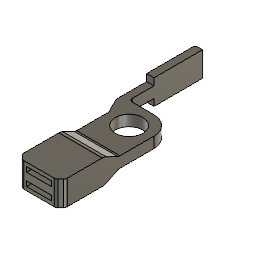
s.piece #1 (Autodesk Fusion 360 design; units mm, degrees)
part number: 2025-12-29-16-31-06-282
Autodesk Fusion 360 part; units mm, degrees
note: some values were not read from the file. Set by a fixed rule: which sketch regions a step uses.
sketch "Sketch1" plane through (0, 0, 0) normal (0, 0, 1) x (1, 0, 0)
  circle A0 centre (0, 0) radius 11
  line L0 (-17.5, -72.5) -> (17.5, -72.5)
  line L1 (17.5, -72.5) -> (17.5, 17.5)
  line L2 (17.5, 17.5) -> (-17.5, 17.5)
  line L3 (-17.5, 17.5) -> (-17.5, -72.5)
  line L4 (-17.5, 76.6964) -> (-17.5, 51.5115)
  line L5 (-17.5, 51.5115) -> (-17.5, 17.5)
  line L6 (-23.5, 76.6964) -> (-23.5, 13.1317)
  line L7 (-23.5, 13.1317) -> (-17.5, 1.0512)
  line L8 (-17.5, 76.6964) -> (-23.5, 76.6964)
  dimension "d1" = 22
  dimension "d2" = 90
  dimension "d3" = 35
  dimension "d4" = 17.5
  dimension "d10" = 17.5
  dimension "d47" = 6
  dimension "d48" = 6
  dimension "d49" = 6
  constraint coincident A0.centre origin
  constraint horizontal L0
  constraint vertical L1
  constraint horizontal L2
  constraint vertical L3
  constraint coincident L2 L3.start
  constraint perpendicular L2 L5
  constraint vertical L6
  constraint coincident L3 L7.end
  constraint perpendicular L6 L8
  measures "d1" diameter of A0
  measures "d2" distance of L0.start L2.end
  measures "d3" distance of L0.start L0.end
  measures "d4" distance of A0.centre L2
  measures "d10" distance of A0.centre L1
  measures "d47" distance of L5 L6
  measures "d48" distance of L3 L6
  measures "d49" distance of L4.start L6.start
extrude "Extrude1" add sketch "Sketch1" along normal blind 20
sketch "Sketch4" plane through (-23.5, 0, 0) normal (-1, 0, 0) x (0, -1, 0)
  line L0 (-1.0512, 0) -> (72.5, 0)
  line L1 (72.5, 0) -> (72.5, 20)
  line L2 (72.5, 20) -> (-1.0512, 20)
  line L3 (72.5, 0) -> (72.5, 20)
  line L4 (37.5, 20) -> (25.7892, 14.3853)
  line L5 (25.7892, 14.3853) -> (-37.5, 14.3853)
  line L6 (-37.5, 14.3853) -> (-37.5, 5.6147)
  line L7 (-37.5, 5.6147) -> (25.7892, 5.6147)
  line L8 (25.7892, 5.6147) -> (37.5, 0)
  line L9 (72.5, 0) -> (72.5, 20)
  line L10 (-17.5, 0) -> (72.5, 0)
  line L11 (37.5, 20) -> (72.5, 20)
  line L12 (72.5, 0) -> (37.5, 0)
  line L13 (-37.5, 14.3853) -> (-37.5, 20)
  line L14 (-1.0512, 20) -> (-1.0512, 0)
  line L15 (-37.5, 0) -> (-37.5, 5.6147)
  line L16 (-1.0512, 20) -> (-1.0512, 0)
  line L17 (-76.6964, 0) -> (-13.1317, 0)
  line L18 (-13.1317, 0) -> (-13.1317, 20)
  line L19 (-13.1317, 20) -> (-76.6964, 20)
  line L20 (-76.6964, 20) -> (-76.6964, 0)
  line L21 (-13.1317, 20) -> (-1.0512, 20)
  dimension "d16" = 110
  dimension "d17" = 35
  dimension "d40" = 5.6147
  dimension "d41" = 8.7705
  constraint coincident L0.end L1.start
  constraint coincident L1.end L2.start
  constraint coincident L2 L4.start
  constraint perpendicular L1 L5
  constraint perpendicular L5 L6
  constraint perpendicular L6 L7
  constraint coincident L0 L8.end
  constraint coincident L2 L13.end
  constraint perpendicular L2 L13
  constraint coincident L2.end L14.start
  constraint coincident L0.start L14.end
  constraint coincident L0 L15.start
  constraint perpendicular L7 L15
  constraint equal L11 L12
  constraint equal L4 L8
  constraint coincident L18.end L19.start
  measures "d16" distance of L6 L9
  measures "d17" distance of L1.end L4.start
  measures "d40" distance of L7 L10
  measures "d41" distance of L5.end L6.end
extrude "Extrude2" cut sketch "Sketch4" against normal blind 52 contours L0 L7 L8 L10 L14 L16 | L7 L10 L14 L16 L18 | L7 L10 L15 L17 L18 | L2 L4 L5 L14 L16 | L5 L14 L16 L18 L21 | L5 L13 L18 L19
chamfer "Chamfer1" distance 4 angle 45 2 edges at (-17.5, -72.5, 10) (17.5, -72.5, 10)
sketch "Sketch6" plane through (0, -72.5, 0) normal (0, -1, 0) x (1, 0, 0)
  line L0 (13.5, 0) -> (13.5, 20)
  line L1 (13.5, 20) -> (-13.5, 20)
  line L2 (-13.5, 20) -> (-13.5, 0)
  line L3 (-13.5, 0) -> (13.5, 0)
  line L4 (-10, 17) -> (10, 17)
  line L5 (10, 13) -> (-10, 13)
  line L6 (-10, 13) -> (-10, 17)
  line L7 (10, 3) -> (10, 7)
  line L8 (10, 7) -> (-10, 7)
  line L9 (-10, 7) -> (-10, 3)
  line L10 (-10, 3) -> (10, 3)
  line L11 (10, 17) -> (10, 13)
  dimension "d25" = 20
  dimension "d26" = 4
  constraint perpendicular L5 L11
  measures "d25" distance of L4.start L4.end
  measures "d26" distance of L4.start L5.end
extrude "Extrude3" cut sketch "Sketch6" against normal blind 30 contours L4 L5 L6 L11 | L7 L8 L9 L10
fillet "Fillet1" radius 4 2 edges at (0, -25.7892, 14.3853) (0, -25.7892, 5.6147)
fillet "Fillet2" radius 7 2 edges at (0, -37.5, 20) (0, -37.5, 0)
fillet "Fillet3" radius 15 1 edges at (17.5, 17.5, 10)
fillet "Fillet4" radius 3 4 edges at (-17.5, -68.5, 10) (-13.5, -72.5, 10) (17.5, -68.5, 10) (13.5, -72.5, 10)
fillet "Fillet6" radius 2.5 3 edges at (-17.5, 1.0512, 10) (-23.5, 13.1317, 10) (-23.5, 76.6964, 10)
fillet "Fillet6" radius 2.5 1 edges at (-17.5, 17.5, 10)
equation "d40 = ( 20 mm - d41 ) / 2"
